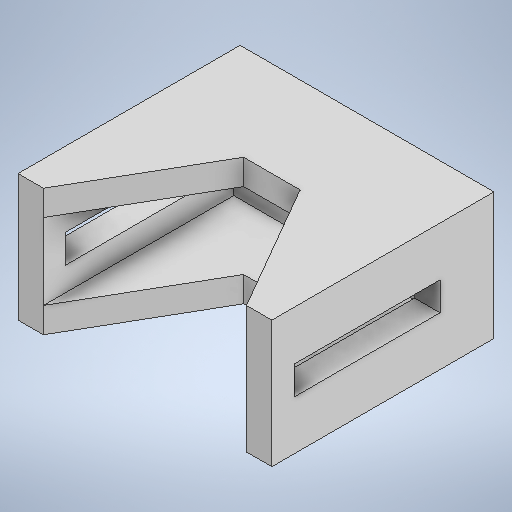
# Autodesk Inventor part: uhelnik_30x30_M4
Saved by Autodesk Inventor 2025 (Build 290162000, 162)
## iProperties
Created: 2025-01-09
Part Number: uhelnik_30x30_M4
Material: Všeobecné
Document SubType Name: Modeling
Designer: lukas
Density: 1 g/cm^3
Appearance: Výchozí
Author: lukas
## iProperties of the stored document uhelnik_30x30_M4_3D tisk.ipt
Created: 2025-01-11
Part Number: uhelnik_30x30_M4_3D tisk
Material: Všeobecné
Document SubType Name: Modeling
Designer: lukas
Density: 1 g/cm^3
Appearance: Výchozí
Author: lukas
Autodesk Inventor part; units mm, degrees
ref_plane "YZ Plane" through (0, 0, 0) normal (1, 0, 0) x (0, 1, 0)
ref_plane "XZ Plane" through (0, 0, 0) normal (0, 1, 0) x (-1, 0, 0)
ref_plane "XY Plane" through (0, 0, 0) normal (0, 0, 1) x (1, 0, 0)
sketch "Náčrt1" plane through (0, 0, 0) normal (0, 0, 1) x (1, 0, 0)
  line L0 (0, 14) -> (0, -14) projected
  line L1 (-28, 0) -> (28, 0) projected
  line L2 (20, -10) -> (-20, -10)
  line L3 (-20, -10) -> (-20, 10)
  line L4 (-20, 10) -> (20, 10)
  line L5 (20, 10) -> (20, -10)
  point P0 (0, 0)
  dimension "d0" = 40
  dimension "d1" = 20
  constraints: 8 end point, 2 parallel, 1 horizontal, 1 perpendicular, 2 other
  measures "d0" distance of L3.end L4.end
  measures "d1" distance between parallel lines of L2 L4
extrude "Vysunutí1" add sketch "Náčrt1" along normal blind 35
sketch "Náčrt2" plane through (0, 0, 35) normal (0, 0, 1) x (1, 0, 0)
  line L0 (20, 10) -> (-20, 10) projected
  line L1 (-20, 10) -> (-20, -10) projected
  line L2 (-20, -10) -> (20, -10) projected
  line L3 (20, -10) -> (20, 10) projected
  line L4 (-16, 6) -> (16, 6)
  line L5 (16, 6) -> (16, -6)
  line L6 (16, -6) -> (-16, -6)
  line L7 (-16, -6) -> (-16, 6)
  point P0 (0, 0)
  dimension "d4" = 4
  constraints: 8 end point, 3 other
  measures "d4" distance between parallel lines of L0 L4
extrude "Vysunutí2" cut sketch "Náčrt2" against normal blind 30 contours L4 L5 L6 L7
sketch "Náčrt3" plane through (0, 0, 5) normal (0, 0, 1) x (1, 0, 0)
  line L0 (16, -6) -> (-16, -6) projected
  line L1 (16, 6) -> (16, -6) projected
  line L2 (-16, 6) -> (16, 6) projected
  line L3 (-16, -6) -> (-16, 6) projected
  line L4 (0, 14) -> (0, -14) projected
  line L5 (-28, 0) -> (28, 0) projected
  line L6 (-5, 2.25) -> (5, 2.25)
  line L7 (5, 2.25) -> (5, -2.25)
  line L8 (5, -2.25) -> (-5, -2.25)
  line L9 (-5, -2.25) -> (-5, 2.25)
  point P0 (0, 0)
  dimension "d7" = 10
  dimension "d8" = 4.5
  constraints: 8 end point, 2 parallel, 1 horizontal, 1 perpendicular, 2 other
  measures "d7" distance of L6.start L6.end
  measures "d8" distance between parallel lines of L8 L6
extrude "Vysunutí3" cut sketch "Náčrt3" against normal through all contours L8 L9 L5 L4 | L4 L5 L7 L8 | L5 L4 L6 L7 | L5 L9 L6 L4
sketch "Náčrt4" plane through (20, -10, 0) normal (1, 0, 0) x (0, 0, -1)
  line L0 (0, 0) -> (0, 20) projected
  line L1 (0, 20) -> (-35, 20) projected
  line L2 (-35, 0) -> (-35, 20) projected
  line L3 (0, 0) -> (-35, 0) projected
  line L4 (-42, 10) -> (7, 10) projected
  line L5 (0, -6) -> (0, 36) projected
  line L6 (-35, 16) -> (-5, 16) projected
  line L7 (-35, 4) -> (-5, 4) projected
  line L8 (-5, 16) -> (-5, 4) projected
  line L9 (-31.5, 7.75) -> (-8.5, 7.75)
  line L10 (-8.5, 7.75) -> (-8.5, 12.25)
  line L11 (-8.5, 12.25) -> (-31.5, 12.25)
  line L12 (-31.5, 12.25) -> (-31.5, 7.75)
  line L13 (-31.5, 10) -> (-8.5, 10)
  line L14 (-8.5, 10) -> (-8.5, 7.75)
  line L15 (-8.5, 7.75) -> (-31.5, 7.75)
  line L16 (-31.5, 7.75) -> (-31.5, 10)
  point P0 (0, 10)
  dimension "d11" = 4.5
  dimension "d12" = 23
  dimension "d13" = 3.5
  constraints: 16 end point, 4 parallel, 2 horizontal, 2 perpendicular, 1 midpoint, 1 other
  measures "d11" distance of L10.end L9.end
  measures "d12" distance of L10.end L11.end
  measures "d13" distance between parallel lines of L10 L8
extrude "Vysunutí4" cut sketch "Náčrt4" against normal through all contours L10 L9 L12 L4 | L4 L12 L11 L10
sketch "Náčrt5" plane through (-20, -10, 0) normal (0, -1, 0) x (1, 0, 0)
  line L0 (0, 0) -> (40, 0) projected
  line L1 (40, 0) -> (40, 35) projected
  line L2 (0, 35) -> (40, 35) projected
  line L3 (0, 0) -> (0, 35) projected
  line L4 (20, 42) -> (20, -7) projected
  line L5 (-8, 0) -> (48, 0) projected
  line L6 (4, 35) -> (4, 5) projected
  line L7 (36, 35) -> (36, 5) projected
  line L8 (4, 35) -> (15.547, 15)
  line L9 (24.453, 15) -> (36, 35)
  line L10 (24.453, 15) -> (15.547, 15)
  line L11 (36, 5) -> (4, 5) projected
  line L12 (4, 35) -> (36, 35)
  point P0 (20, 0)
  dimension "d16" = 30
  dimension "d17" = 30
  dimension "d18" = 10
  constraints: 8 end point, 2 perpendicular
  measures "d16" angle of L7 L9
  measures "d17" angle of L6 L8
  measures "d18" distance between parallel lines of L10 L11
extrude "Vysunutí5" cut sketch "Náčrt5" against normal through all contours L2 L4 L10 L8 | L4 L2 L9 L10
